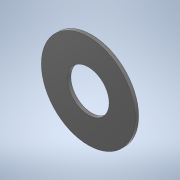
# Autodesk Inventor part: UUW-0614-05BH
Saved by Autodesk Inventor 2020.4 (Build 244396000, 396)
## iProperties
Part Number: UUW-0614-05BH
Material: ステンレス鋼 AISI 304
Document SubType Name: Modeling
Designer: Masato Kubotera
Density: 7.221 g/cm^3
Appearance: 滑らか - 黒
Mass: 0.44679 g
Surface Area: 2.79225 cm^2
Volume: 0.0618737 cm^3
Description: ReadyMade
Catalog Web Link: https://www.hirosugi-net.co.jp/shop/g/g59960/
Author: Masato Kubotera
Autodesk Inventor part; units mm, degrees
ref_plane "YZ Plane" through (0, 0, 0) normal (1, 0, 0) x (0, 1, 0)
ref_plane "XZ Plane" through (0, 0, 0) normal (0, 1, 0) x (-1, 0, 0)
ref_plane "XY Plane" through (0, 0, 0) normal (0, 0, 1) x (1, 0, 0)
sketch "スケッチ1" plane through (0, 0, 0) normal (0, 0, 1) x (1, 0, 0)
  circle A0 centre (0, 0) radius 3.1
  circle A1 centre (0, 0) radius 7
  dimension "d0" = 6.2
  dimension "d1" = 14
  constraints: 2 centre point, 2 coincident
  measures "d0" diameter of A0
  measures "d1" diameter of A1
extrude "押し出し1" add sketch "スケッチ1" along normal blind 0.5
